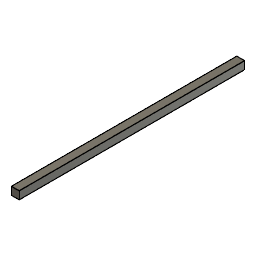
Beam_600mm (Autodesk Fusion 360 design; units mm, degrees)
part number: 2026-09-01-20-19-48-186
Autodesk Fusion 360 part; units mm, degrees
sketch "Sketch1" plane through (0, 0, 0) normal (0, 0, 1) x (1, 0, 0)
  line L0 (-10.5, -10.5) -> (10.5, -10.5)
  line L1 (10.5, -10.5) -> (10.5, 10.5)
  line L2 (10.5, 10.5) -> (-10.5, 10.5)
  line L3 (-10.5, 10.5) -> (-10.5, -10.5)
extrude "Extrude1" add sketch "Sketch1" along normal blind 600
sketch "Sketch2" plane through (0, 0, 0) normal (0, 1, 0) x (1, 0, 0)
  circle A0 centre (0, 10.28) radius 6.25
sketch "Sketch3" plane through (0, 0, 0) normal (0, 1, 0) x (1, 0, 0)
  circle A0 centre (0, 589.72) radius 6.25
sketch "Sketch4" plane through (0, 0, 0) normal (0, 1, 0) x (1, 0, 0)
  circle A0 centre (0, 10.28) radius 6.25
sketch "Sketch5" plane through (0, 0, 0) normal (0, 1, 0) x (1, 0, 0)
  circle A0 centre (0, 589.72) radius 6.25
sketch "Sketch6" plane through (0, 0, 0) normal (1, 0, 0) x (0, 0, -1)
  circle A0 centre (0, 10.28) radius 6.25
sketch "Sketch7" plane through (0, 0, 0) normal (1, 0, 0) x (0, 0, -1)
  circle A0 centre (0, 589.72) radius 6.25
named bodies: "Beam_A500"
